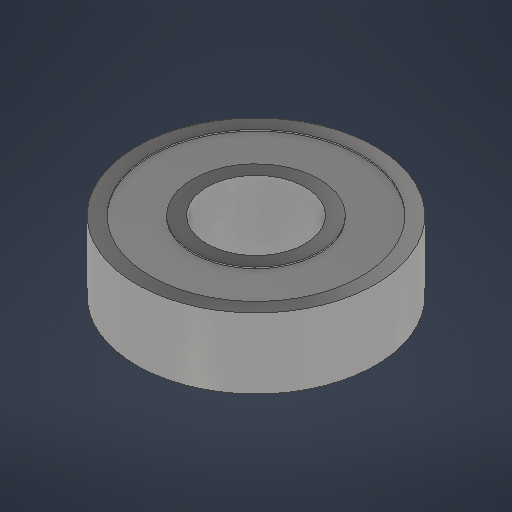
# Autodesk Inventor part: Kugellager 14 x 7 x 5
Saved by Autodesk Inventor 2025.2 (Build 292293000, 293)
## iProperties
Created: 2024-11-07
Part Number: Kugellager 14 x 7 x 5
Material: Generisch
Document SubType Name: Modeling
Designer: Fabian
Density: 1 g/cm^3
Appearance: Vorgabe
Author: Fabian
Autodesk Inventor part; units mm, degrees
ref_plane "YZ Plane" through (0, 0, 0) normal (1, 0, 0) x (0, 1, 0)
ref_plane "XZ Plane" through (0, 0, 0) normal (0, 1, 0) x (-1, 0, 0)
ref_plane "XY Plane" through (0, 0, 0) normal (0, 0, 1) x (1, 0, 0)
sketch "Skizze1" plane through (0, 0, 0) normal (0, 1, 0) x (-1, 0, 0)
  circle A0 centre (0, 0) radius 8.5
  circle A1 centre (0, 0) radius 3.5
  circle A2 centre (0, 0) radius 7.5
  circle A3 centre (0, 0) radius 4.5
  dimension "d0" = 17
  dimension "d1" = 7
  dimension "d2" = 1
  dimension "d3" = 1
  constraints: 4 centre point, 2 coincident
  measures "d0" diameter of A0
  measures "d1" diameter of A1
  measures "d2" radial gap between concentric circles of A0 A2
  measures "d3" radial gap between concentric circles of A1 A3
extrude "Extrusion1" add sketch "Skizze1" along normal mid plane 5
extrude "Extrusion2" add sketch "Skizze1" along normal mid plane 4.8 contours A2
